Autodesk Fusion 360 part; units mm, degrees
(part 6 of 6)
  spline S11 degree 5 poles (-54.7383, -24.4894) (-54.7257, -24.481) (-54.7005, -24.464) (-54.6628, -24.4385) (-54.6128, -24.4043) (-54.5506, -24.3613) (-54.4888, -24.3181) (-54.4272, -24.2746) (-54.366, -24.2308) (-54.3052, -24.1868) (-54.2446, -24.1425) (-54.1845, -24.098) (-54.1246, -24.0531) (-54.0651, -24.0081) (-54.006, -23.9627) (-53.9472, -23.9171) (-53.8888, -23.8713) (-53.8308, -23.8252) (-53.7731, -23.7788) (-53.7158, -23.7322) (-53.6588, -23.6853) (-53.6023, -23.6381) (-53.5461, -23.5907) (-53.4903, -23.543) (-53.4349, -23.4951) (-53.3798, -23.4469) (-53.3252, -23.3985) (-53.271, -23.3498) (-53.2171, -23.3008) (-53.1637, -23.2516) (-53.1107, -23.2021) (-53.0581, -23.1524) (-53.006, -23.1024) (-52.9543, -23.0522) (-52.903, -23.0017) (-52.8521, -22.9509) (-52.8017, -22.8999) (-52.7517, -22.8486) (-52.7022, -22.797) (-52.6531, -22.7452) (-52.6046, -22.6931) (-52.5565, -22.6408) (-52.5088, -22.5882) (-52.4617, -22.5353) (-52.4151, -22.4822) (-52.369, -22.4288) (-52.3234, -22.3751) (-52.2783, -22.3212) (-52.2337, -22.267) (-52.1896, -22.2126) (-52.1461, -22.1579) (-52.1033, -22.1028) (-52.061, -22.0475) (-52.0194, -21.9919) (-51.9783, -21.936) (-51.9379, -21.8799) (-51.8981, -21.8234) (-51.8587, -21.7667) (-51.82, -21.7098) (-51.782, -21.6526) (-51.7447, -21.595) (-51.7084, -21.537) (-51.6732, -21.4786) (-51.6389, -21.4198) (-51.6056, -21.3607) (-51.5729, -21.3012) (-51.5407, -21.2416) (-51.5091, -21.1818) (-51.4781, -21.1218) (-51.4485, -21.0613) (-51.421, -21) (-51.4013, -20.9502) (-51.3882, -20.9122) (-51.3802, -20.8866) (-51.3764, -20.8737) knots -1 -1 -1 -1 -1 -1 -0.98571429 -0.97142857 -0.95714286 -0.94285714 -0.92857143 -0.91428571 -0.9 -0.88571429 -0.87142857 -0.85714286 -0.84285714 -0.82857143 -0.81428571 -0.8 -0.78571429 -0.77142857 -0.75714286 -0.74285714 -0.72857143 -0.71428571 -0.7 -0.68571429 -0.67142857 -0.65714286 -0.64285714 -0.62857143 -0.61428571 -0.6 -0.58571429 -0.57142857 -0.55714286 -0.54285714 -0.52857143 -0.51428571 -0.5 -0.48571429 -0.47142857 -0.45714286 -0.44285714 -0.42857143 -0.41428571 -0.4 -0.38571429 -0.37142857 -0.35714286 -0.34285714 -0.32857143 -0.31428571 -0.3 -0.28571429 -0.27142857 -0.25714286 -0.24285714 -0.22857143 -0.21428571 -0.2 -0.18571429 -0.17142857 -0.15714286 -0.14285714 -0.12857143 -0.11428571 -0.1 -0.08571429 -0.07142857 -0.05714286 -0.04285714 -0.02857143 -0.01428571 0 0 0 0 0 0
  line L13 (-51.3764, -20.8737) -> (-51.0935, -19.9176)
  arc A22 (-49.2442, -18.8145) -> (-51.0935, -19.9176) centre (-49.5712, -20.368) ccw
  arc A23 (-49.2442, -18.8145) -> (-48.5053, -18.9543) centre (-45.4614, -0.8441) ccw
  arc A24 (-47.1869, -20.6568) -> (-48.5053, -18.9543) centre (-48.7685, -20.5199) ccw
  line L14 (-47.1869, -20.6568) -> (-47.2729, -21.6501)
  spline S12 degree 5 poles (-47.2729, -21.6501) (-47.274, -21.6635) (-47.2759, -21.6902) (-47.2776, -21.7304) (-47.2775, -21.784) (-47.2743, -21.8511) (-47.2688, -21.9182) (-47.2619, -21.9854) (-47.2543, -22.0527) (-47.2461, -22.1199) (-47.2375, -22.1872) (-47.228, -22.2544) (-47.2176, -22.3217) (-47.2061, -22.3889) (-47.1935, -22.4561) (-47.1799, -22.5233) (-47.1654, -22.5905) (-47.1501, -22.6577) (-47.1342, -22.7248) (-47.1177, -22.7919) (-47.1006, -22.8589) (-47.0829, -22.9259) (-47.0644, -22.9929) (-47.0453, -23.0599) (-47.0255, -23.1267) (-47.005, -23.1936) (-46.9839, -23.2604) (-46.9622, -23.3271) (-46.9399, -23.3938) (-46.917, -23.4604) (-46.8936, -23.5269) (-46.8696, -23.5934) (-46.8451, -23.6598) (-46.82, -23.7262) (-46.7943, -23.7925) (-46.7681, -23.8587) (-46.7414, -23.9249) (-46.7141, -23.9909) (-46.6863, -24.0569) (-46.658, -24.1229) (-46.6292, -24.1887) (-46.5999, -24.2545) (-46.5702, -24.3201) (-46.5399, -24.3857) (-46.5091, -24.4512) (-46.4778, -24.5167) (-46.4461, -24.582) (-46.4139, -24.6472) (-46.3812, -24.7124) (-46.348, -24.7774) (-46.3144, -24.8424) (-46.2803, -24.9072) (-46.2458, -24.972) (-46.2108, -25.0367) (-46.1754, -25.1012) (-46.1395, -25.1657) (-46.1032, -25.23) (-46.0664, -25.2943) (-46.0292, -25.3584) (-45.9916, -25.4224) (-45.9536, -25.4863) (-45.9151, -25.5501) (-45.8762, -25.6138) (-45.8369, -25.6774) (-45.7971, -25.7409) (-45.757, -25.8042) (-45.7164, -25.8674) (-45.6754, -25.9305) (-45.634, -25.9935) (-45.5922, -26.0564) (-45.55, -26.1191) (-45.516, -26.1692) (-45.4902, -26.2067) (-45.473, -26.2317) (-45.4643, -26.2441) knots 0 0 0 0 0 0 0.01428571 0.02857143 0.04285714 0.05714286 0.07142857 0.08571429 0.1 0.11428571 0.12857143 0.14285714 0.15714286 0.17142857 0.18571429 0.2 0.21428571 0.22857143 0.24285714 0.25714286 0.27142857 0.28571429 0.3 0.31428571 0.32857143 0.34285714 0.35714286 0.37142857 0.38571429 0.4 0.41428571 0.42857143 0.44285714 0.45714286 0.47142857 0.48571429 0.5 0.51428571 0.52857143 0.54285714 0.55714286 0.57142857 0.58571429 0.6 0.61428571 0.62857143 0.64285714 0.65714286 0.67142857 0.68571429 0.7 0.71428571 0.72857143 0.74285714 0.75714286 0.77142857 0.78571429 0.8 0.81428571 0.82857143 0.84285714 0.85714286 0.87142857 0.88571429 0.9 0.91428571 0.92857143 0.94285714 0.95714286 0.97142857 0.98571429 1 1 1 1 1 1
  arc A25 (-45.4643, -26.2441) -> (-43.5603, -26.1729) centre (-45.4614, -0.8441) ccw
  spline S13 degree 5 poles (-43.5603, -26.1729) (-43.5526, -26.1598) (-43.5373, -26.1336) (-43.5144, -26.0943) (-43.4842, -26.0418) (-43.4468, -25.9761) (-43.4098, -25.9103) (-43.3732, -25.8444) (-43.3371, -25.7784) (-43.3013, -25.7123) (-43.266, -25.6462) (-43.2311, -25.5799) (-43.1967, -25.5136) (-43.1626, -25.4471) (-43.129, -25.3806) (-43.0959, -25.3141) (-43.0631, -25.2474) (-43.0308, -25.1807) (-42.999, -25.1139) (-42.9676, -25.047) (-42.9366, -24.98) (-42.9061, -24.913) (-42.8761, -24.8459) (-42.8465, -24.7788) (-42.8173, -24.7115) (-42.7887, -24.6442) (-42.7605, -24.5769) (-42.7327, -24.5095) (-42.7055, -24.442) (-42.6787, -24.3745) (-42.6524, -24.3069) (-42.6266, -24.2393) (-42.6013, -24.1716) (-42.5765, -24.1039) (-42.5522, -24.0362) (-42.5284, -23.9683) (-42.5052, -23.9005) (-42.4824, -23.8326) (-42.4601, -23.7647) (-42.4384, -23.6967) (-42.4172, -23.6287) (-42.3966, -23.5607) (-42.3765, -23.4926) (-42.357, -23.4246) (-42.3381, -23.3565) (-42.3197, -23.2884) (-42.3019, -23.2202) (-42.2846, -23.1521) (-42.268, -23.0839) (-42.2519, -23.0157) (-42.2365, -22.9475) (-42.2217, -22.8794) (-42.2076, -22.8112) (-42.1942, -22.743) (-42.1815, -22.6749) (-42.1695, -22.6067) (-42.1581, -22.5386) (-42.1472, -22.4705) (-42.137, -22.4024) (-42.1276, -22.3343) (-42.119, -22.2663) (-42.1115, -22.1983) (-42.105, -22.1304) (-42.0997, -22.0625) (-42.0953, -21.9948) (-42.0917, -21.927) (-42.0886, -21.8594) (-42.086, -21.7918) (-42.0841, -21.7242) (-42.0837, -21.6569) (-42.0855, -21.5897) (-42.0894, -21.5363) (-42.0941, -21.4963) (-42.098, -21.4698) (-42.1001, -21.4566) knots -1 -1 -1 -1 -1 -1 -0.98571429 -0.97142857 -0.95714286 -0.94285714 -0.92857143 -0.91428571 -0.9 -0.88571429 -0.87142857 -0.85714286 -0.84285714 -0.82857143 -0.81428571 -0.8 -0.78571429 -0.77142857 -0.75714286 -0.74285714 -0.72857143 -0.71428571 -0.7 -0.68571429 -0.67142857 -0.65714286 -0.64285714 -0.62857143 -0.61428571 -0.6 -0.58571429 -0.57142857 -0.55714286 -0.54285714 -0.52857143 -0.51428571 -0.5 -0.48571429 -0.47142857 -0.45714286 -0.44285714 -0.42857143 -0.41428571 -0.4 -0.38571429 -0.37142857 -0.35714286 -0.34285714 -0.32857143 -0.31428571 -0.3 -0.28571429 -0.27142857 -0.25714286 -0.24285714 -0.22857143 -0.21428571 -0.2 -0.18571429 -0.17142857 -0.15714286 -0.14285714 -0.12857143 -0.11428571 -0.1 -0.08571429 -0.07142857 -0.05714286 -0.04285714 -0.02857143 -0.01428571 0 0 0 0 0 0
  line L15 (-42.1001, -21.4566) -> (-42.2601, -20.4724)
  arc A26 (-41.0726, -18.6762) -> (-42.2601, -20.4724) centre (-40.6932, -20.2177) ccw
  arc A27 (-41.0726, -18.6762) -> (-40.3462, -18.4816) centre (-45.4614, -0.8441) ccw
  arc A28 (-38.4196, -19.4434) -> (-40.3462, -18.4816) centre (-39.904, -20.0062) ccw
  line L16 (-38.4196, -19.4434) -> (-38.0661, -20.3756)
  spline S14 degree 5 poles (-38.0661, -20.3756) (-38.0613, -20.3882) (-38.0515, -20.4131) (-38.0355, -20.45) (-38.0122, -20.4983) (-37.9802, -20.5573) (-37.9461, -20.6155) (-37.9108, -20.673) (-37.8747, -20.7303) (-37.8382, -20.7873) (-37.8012, -20.8441) (-37.7635, -20.9006) (-37.725, -20.9567) (-37.6854, -21.0123) (-37.6449, -21.0674) (-37.6034, -21.122) (-37.5612, -21.1763) (-37.5183, -21.2302) (-37.4749, -21.2837) (-37.4309, -21.337) (-37.3864, -21.39) (-37.3414, -21.4427) (-37.2957, -21.495) (-37.2494, -21.547) (-37.2025, -21.5987) (-37.1551, -21.65) (-37.1071, -21.701) (-37.0586, -21.7517) (-37.0095, -21.8021) (-36.96, -21.8522) (-36.9101, -21.902) (-36.8596, -21.9515) (-36.8087, -22.0007) (-36.7573, -22.0496) (-36.7054, -22.0982) (-36.653, -22.1465) (-36.6003, -22.1945) (-36.547, -22.2422) (-36.4934, -22.2896) (-36.4393, -22.3368) (-36.3848, -22.3836) (-36.3298, -22.4301) (-36.2745, -22.4764) (-36.2187, -22.5223) (-36.1626, -22.568) (-36.106, -22.6134) (-36.0491, -22.6585) (-35.9918, -22.7033) (-35.9341, -22.7478) (-35.876, -22.792) (-35.8175, -22.8359) (-35.7586, -22.8796) (-35.6994, -22.9229) (-35.6399, -22.966) (-35.5799, -23.0088) (-35.5196, -23.0513) (-35.459, -23.0935) (-35.398, -23.1355) (-35.3367, -23.1771) (-35.275, -23.2185) (-35.213, -23.2595) (-35.1506, -23.3003) (-35.0879, -23.3408) (-35.0249, -23.3811) (-34.9616, -23.421) (-34.8979, -23.4606) (-34.8339, -23.5) (-34.7696, -23.5391) (-34.705, -23.5778) (-34.6401, -23.6163) (-34.5749, -23.6545) (-34.5224, -23.6849) (-34.483, -23.7075) (-34.4566, -23.7225) (-34.4434, -23.73) knots 0 0 0 0 0 0 0.01428571 0.02857143 0.04285714 0.05714286 0.07142857 0.08571429 0.1 0.11428571 0.12857143 0.14285714 0.15714286 0.17142857 0.18571429 0.2 0.21428571 0.22857143 0.24285714 0.25714286 0.27142857 0.28571429 0.3 0.31428571 0.32857143 0.34285714 0.35714286 0.37142857 0.38571429 0.4 0.41428571 0.42857143 0.44285714 0.45714286 0.47142857 0.48571429 0.5 0.51428571 0.52857143 0.54285714 0.55714286 0.57142857 0.58571429 0.6 0.61428571 0.62857143 0.64285714 0.65714286 0.67142857 0.68571429 0.7 0.71428571 0.72857143 0.74285714 0.75714286 0.77142857 0.78571429 0.8 0.81428571 0.82857143 0.84285714 0.85714286 0.87142857 0.88571429 0.9 0.91428571 0.92857143 0.94285714 0.95714286 0.97142857 0.98571429 1 1 1 1 1 1
  arc A29 (-34.4434, -23.73) -> (-32.7588, -22.8397) centre (-45.4614, -0.8441) ccw
  spline S15 degree 5 poles (-32.7588, -22.8397) (-32.7576, -22.8246) (-32.7551, -22.7943) (-32.7516, -22.749) (-32.7471, -22.6886) (-32.7419, -22.6131) (-32.7372, -22.5378) (-32.7328, -22.4626) (-32.7289, -22.3874) (-32.7254, -22.3124) (-32.7223, -22.2375) (-32.7196, -22.1626) (-32.7173, -22.0879) (-32.7154, -22.0133) (-32.714, -21.9388) (-32.713, -21.8644) (-32.7125, -21.7902) (-32.7123, -21.716) (-32.7126, -21.642) (-32.7133, -21.5681) (-32.7145, -21.4944) (-32.7161, -21.4208) (-32.7181, -21.3473) (-32.7206, -21.2739) (-32.7235, -21.2007) (-32.7269, -21.1277) (-32.7307, -21.0547) (-32.735, -20.982) (-32.7397, -20.9094) (-32.7448, -20.8369) (-32.7505, -20.7646) (-32.7566, -20.6925) (-32.7631, -20.6206) (-32.7702, -20.5488) (-32.7777, -20.4772) (-32.7857, -20.4058) (-32.7941, -20.3345) (-32.8031, -20.2635) (-32.8125, -20.1926) (-32.8224, -20.122) (-32.8328, -20.0515) (-32.8438, -19.9813) (-32.8552, -19.9113) (-32.8672, -19.8415) (-32.8796, -19.7719) (-32.8926, -19.7026) (-32.9062, -19.6334) (-32.9202, -19.5646) (-32.9347, -19.4959) (-32.9499, -19.4275) (-32.9655, -19.3594) (-32.9818, -19.2916) (-32.9987, -19.224) (-33.0162, -19.1568) (-33.0343, -19.0899) (-33.0531, -19.0233) (-33.0723, -18.9569) (-33.0921, -18.8908) (-33.1125, -18.8251) (-33.1335, -18.7596) (-33.1553, -18.6946) (-33.178, -18.6301) (-33.2017, -18.5661) (-33.2263, -18.5027) (-33.2517, -18.4397) (-33.2778, -18.3771) (-33.3044, -18.3148) (-33.3314, -18.2528) (-33.3591, -18.1911) (-33.3879, -18.1302) (-33.4186, -18.0705) (-33.4453, -18.0241) (-33.4669, -17.9901) (-33.4819, -17.9679) (-33.4896, -17.9569) knots -1 -1 -1 -1 -1 -1 -0.98571429 -0.97142857 -0.95714286 -0.94285714 -0.92857143 -0.91428571 -0.9 -0.88571429 -0.87142857 -0.85714286 -0.84285714 -0.82857143 -0.81428571 -0.8 -0.78571429 -0.77142857 -0.75714286 -0.74285714 -0.72857143 -0.71428571 -0.7 -0.68571429 -0.67142857 -0.65714286 -0.64285714 -0.62857143 -0.61428571 -0.6 -0.58571429 -0.57142857 -0.55714286 -0.54285714 -0.52857143 -0.51428571 -0.5 -0.48571429 -0.47142857 -0.45714286 -0.44285714 -0.42857143 -0.41428571 -0.4 -0.38571429 -0.37142857 -0.35714286 -0.34285714 -0.32857143 -0.31428571 -0.3 -0.28571429 -0.27142857 -0.25714286 -0.24285714 -0.22857143 -0.21428571 -0.2 -0.18571429 -0.17142857 -0.15714286 -0.14285714 -0.12857143 -0.11428571 -0.1 -0.08571429 -0.07142857 -0.05714286 -0.04285714 -0.02857143 -0.01428571 0 0 0 0 0 0
  line L17 (-33.4896, -17.9569) -> (-34.0607, -17.1396)
  arc A30 (-33.7702, -15.006) -> (-34.0607, -17.1396) centre (-32.7595, -16.2303) ccw
  arc A31 (-33.7702, -15.006) -> (-33.2001, -14.5155) centre (-45.4614, -0.8441) ccw
  arc A32 (-31.0471, -14.5462) -> (-33.2001, -14.5155) centre (-32.1402, -15.6973) ccw
  line L18 (-31.0471, -14.5462) -> (-30.3241, -15.2327)
  spline S16 degree 5 poles (-30.3241, -15.2327) (-30.3143, -15.242) (-30.2946, -15.2602) (-30.2642, -15.2865) (-30.2223, -15.3199) (-30.1678, -15.3592) (-30.1119, -15.3967) (-30.0551, -15.4332) (-29.9978, -15.4692) (-29.9401, -15.5048) (-29.8821, -15.5399) (-29.8236, -15.5744) (-29.7646, -15.6082) (-29.7048, -15.6412) (-29.6444, -15.6732) (-29.5834, -15.7045) (-29.5218, -15.735) (-29.4598, -15.765) (-29.3974, -15.7944) (-29.3347, -15.8233) (-29.2716, -15.8518) (-29.2081, -15.8797) (-29.1443, -15.907) (-29.08, -15.9338) (-29.0153, -15.96) (-28.9503, -15.9856) (-28.8849, -16.0108) (-28.8192, -16.0354) (-28.7532, -16.0595) (-28.6869, -16.0832) (-28.6202, -16.1064) (-28.5533, -16.1291) (-28.4861, -16.1513) (-28.4185, -16.1731) (-28.3507, -16.1943) (-28.2826, -16.2151) (-28.2142, -16.2355) (-28.1455, -16.2554) (-28.0766, -16.2748) (-28.0074, -16.2938) (-27.938, -16.3123) (-27.8683, -16.3304) (-27.7984, -16.3481) (-27.7282, -16.3653) (-27.6578, -16.3821) (-27.5872, -16.3984) (-27.5163, -16.4143) (-27.4452, -16.4298) (-27.3739, -16.4449) (-27.3024, -16.4595) (-27.2307, -16.4737) (-27.1587, -16.4875) (-27.0865, -16.5009) (-27.0142, -16.5139) (-26.9416, -16.5264) (-26.8689, -16.5386) (-26.7959, -16.5503) (-26.7228, -16.5616) (-26.6494, -16.5725) (-26.5759, -16.583) (-26.5022, -16.5931) (-26.4283, -16.6028) (-26.3543, -16.6121) (-26.2801, -16.621) (-26.2057, -16.6295) (-26.1311, -16.6376) (-26.0564, -16.6453) (-25.9815, -16.6526) (-25.9065, -16.6595) (-25.8313, -16.666) (-25.7559, -16.6721) (-25.6955, -16.6767) (-25.6501, -16.68) (-25.6199, -16.6821) (-25.6047, -16.6831) knots 0 0 0 0 0 0 0.01428571 0.02857143 0.04285714 0.05714286 0.07142857 0.08571429 0.1 0.11428571 0.12857143 0.14285714 0.15714286 0.17142857 0.18571429 0.2 0.21428571 0.22857143 0.24285714 0.25714286 0.27142857 0.28571429 0.3 0.31428571 0.32857143 0.34285714 0.35714286 0.37142857 0.38571429 0.4 0.41428571 0.42857143 0.44285714 0.45714286 0.47142857 0.48571429 0.5 0.51428571 0.52857143 0.54285714 0.55714286 0.57142857 0.58571429 0.6 0.61428571 0.62857143 0.64285714 0.65714286 0.67142857 0.68571429 0.7 0.71428571 0.72857143 0.74285714 0.75714286 0.77142857 0.78571429 0.8 0.81428571 0.82857143 0.84285714 0.85714286 0.87142857 0.88571429 0.9 0.91428571 0.92857143 0.94285714 0.95714286 0.97142857 0.98571429 1 1 1 1 1 1
  arc A33 (-25.6047, -16.6831) -> (-24.4732, -15.15) centre (-45.4614, -0.8441) ccw
  spline S17 degree 5 poles (-24.4732, -15.15) (-24.4787, -15.1359) (-24.4896, -15.1075) (-24.5061, -15.0651) (-24.5283, -15.0088) (-24.5564, -14.9386) (-24.5847, -14.8686) (-24.6135, -14.799) (-24.6425, -14.7296) (-24.6719, -14.6604) (-24.7016, -14.5916) (-24.7317, -14.523) (-24.762, -14.4547) (-24.7927, -14.3866) (-24.8238, -14.3189) (-24.8552, -14.2515) (-24.8869, -14.1843) (-24.9189, -14.1175) (-24.9513, -14.0509) (-24.984, -13.9846) (-25.017, -13.9187) (-25.0504, -13.8531) (-25.0841, -13.7877) (-25.1182, -13.7227) (-25.1526, -13.658) (-25.1873, -13.5937) (-25.2224, -13.5296) (-25.2578, -13.4659) (-25.2935, -13.4025) (-25.3296, -13.3395) (-25.3661, -13.2768) (-25.4029, -13.2145) (-25.44, -13.1525) (-25.4775, -13.0909) (-25.5153, -13.0297) (-25.5535, -12.9688) (-25.592, -12.9083) (-25.6309, -12.8481) (-25.6701, -12.7884) (-25.7097, -12.729) (-25.7497, -12.6701) (-25.79, -12.6115) (-25.8307, -12.5534) (-25.8718, -12.4957) (-25.9132, -12.4385) (-25.955, -12.3816) (-25.9971, -12.3252) (-26.0397, -12.2692) (-26.0826, -12.2137) (-26.1259, -12.1586) (-26.1695, -12.1041) (-26.2136, -12.05) (-26.2582, -11.9965) (-26.3031, -11.9435) (-26.3485, -11.8911) (-26.3942, -11.8392) (-26.4404, -11.7878) (-26.4869, -11.7368) (-26.5338, -11.6864) (-26.5811, -11.6366) (-26.629, -11.5875) (-26.6774, -11.5392) (-26.7265, -11.4918) (-26.7762, -11.4453) (-26.8265, -11.3996) (-26.8771, -11.3546) (-26.9281, -11.3099) (-26.9793, -11.2658) (-27.031, -11.2222) (-27.0834, -11.1799) (-27.137, -11.1394) (-27.1812, -11.1092) (-27.2153, -11.0879) (-27.2385, -11.0744) (-27.2502, -11.0678) knots -1 -1 -1 -1 -1 -1 -0.98571429 -0.97142857 -0.95714286 -0.94285714 -0.92857143 -0.91428571 -0.9 -0.88571429 -0.87142857 -0.85714286 -0.84285714 -0.82857143 -0.81428571 -0.8 -0.78571429 -0.77142857 -0.75714286 -0.74285714 -0.72857143 -0.71428571 -0.7 -0.68571429 -0.67142857 -0.65714286 -0.64285714 -0.62857143 -0.61428571 -0.6 -0.58571429 -0.57142857 -0.55714286 -0.54285714 -0.52857143 -0.51428571 -0.5 -0.48571429 -0.47142857 -0.45714286 -0.44285714 -0.42857143 -0.41428571 -0.4 -0.38571429 -0.37142857 -0.35714286 -0.34285714 -0.32857143 -0.31428571 -0.3 -0.28571429 -0.27142857 -0.25714286 -0.24285714 -0.22857143 -0.21428571 -0.2 -0.18571429 -0.17142857 -0.15714286 -0.14285714 -0.12857143 -0.11428571 -0.1 -0.08571429 -0.07142857 -0.05714286 -0.04285714 -0.02857143 -0.01428571 0 0 0 0 0 0
  line L19 (-27.2502, -11.0678) -> (-28.1194, -10.5793)
  arc A34 (-28.7833, -8.5309) -> (-28.1194, -10.5793) centre (-27.3416, -9.1954) ccw
  arc A35 (-28.7833, -8.5309) -> (-28.4826, -7.8417) centre (-45.4614, -0.8441) ccw
  arc A36 (-26.5294, -6.9351) -> (-28.4826, -7.8417) centre (-27.0149, -8.4466) ccw
  line L20 (-26.5294, -6.9351) -> (-25.5802, -7.24)
  spline S18 degree 5 poles (-25.5802, -7.24) (-25.5674, -7.2441) (-25.5417, -7.2519) (-25.5029, -7.2625) (-25.4506, -7.2743) (-25.3845, -7.2861) (-25.3178, -7.2957) (-25.2508, -7.3039) (-25.1836, -7.3115) (-25.1162, -7.3185) (-25.0487, -7.325) (-24.981, -7.3307) (-24.9131, -7.3356) (-24.845, -7.3393) (-24.7767, -7.342) (-24.7081, -7.3436) (-24.6394, -7.3444) (-24.5705, -7.3445) (-24.5016, -7.344) (-24.4325, -7.3428) (-24.3633, -7.3411) (-24.294, -7.3387) (-24.2246, -7.3356) (-24.1551, -7.3318) (-24.0855, -7.3274) (-24.0158, -7.3223) (-23.946, -7.3165) (-23.8761, -7.3102) (-23.8061, -7.3033) (-23.7361, -7.2959) (-23.666, -7.2878) (-23.5958, -7.2793) (-23.5256, -7.2701) (-23.4553, -7.2604) (-23.385, -7.2501) (-23.3146, -7.2393) (-23.2442, -7.228) (-23.1737, -7.2161) (-23.1031, -7.2037) (-23.0326, -7.1908) (-22.962, -7.1774) (-22.8914, -7.1635) (-22.8207, -7.149) (-22.75, -7.1341) (-22.6793, -7.1187) (-22.6086, -7.1027) (-22.5378, -7.0863) (-22.467, -7.0694) (-22.3962, -7.0521) (-22.3254, -7.0342) (-22.2546, -7.0159) (-22.1838, -6.9971) (-22.113, -6.9779) (-22.0422, -6.9581) (-21.9714, -6.938) (-21.9005, -6.9173) (-21.8297, -6.8962) (-21.7589, -6.8747) (-21.6881, -6.8527) (-21.6173, -6.8303) (-21.5465, -6.8074) (-21.4758, -6.7841) (-21.405, -6.7603) (-21.3343, -6.7361) (-21.2636, -6.7115) (-21.1929, -6.6865) (-21.1222, -6.661) (-21.0516, -6.6351) (-20.981, -6.6087) (-20.9104, -6.582) (-20.8399, -6.5548) (-20.7834, -6.5327) (-20.7412, -6.516) (-20.713, -6.5047) (-20.6989, -6.4991) knots 0 0 0 0 0 0 0.01428571 0.02857143 0.04285714 0.05714286 0.07142857 0.08571429 0.1 0.11428571 0.12857143 0.14285714 0.15714286 0.17142857 0.18571429 0.2 0.21428571 0.22857143 0.24285714 0.25714286 0.27142857 0.28571429 0.3 0.31428571 0.32857143 0.34285714 0.35714286 0.37142857 0.38571429 0.4 0.41428571 0.42857143 0.44285714 0.45714286 0.47142857 0.48571429 0.5 0.51428571 0.52857143 0.54285714 0.55714286 0.57142857 0.58571429 0.6 0.61428571 0.62857143 0.64285714 0.65714286 0.67142857 0.68571429 0.7 0.71428571 0.72857143 0.74285714 0.75714286 0.77142857 0.78571429 0.8 0.81428571 0.82857143 0.84285714 0.85714286 0.87142857 0.88571429 0.9 0.91428571 0.92857143 0.94285714 0.95714286 0.97142857 0.98571429 1 1 1 1 1 1
  arc A37 (-20.6989, -6.4991) -> (-20.3446, -4.6269) centre (-45.4614, -0.8441) ccw
  spline S19 degree 5 poles (-20.3446, -4.6269) (-20.3557, -4.6165) (-20.3778, -4.5957) (-20.4111, -4.5647) (-20.4555, -4.5235) (-20.5113, -4.4724) (-20.5672, -4.4217) (-20.6233, -4.3714) (-20.6796, -4.3215) (-20.736, -4.272) (-20.7927, -4.2228) (-20.8495, -4.1741) (-20.9065, -4.1257) (-20.9637, -4.0777) (-21.0211, -4.0302) (-21.0786, -3.983) (-21.1363, -3.9363) (-21.1942, -3.8899) (-21.2522, -3.844) (-21.3104, -3.7985) (-21.3688, -3.7534) (-21.4274, -3.7088) (-21.4861, -3.6645) (-21.545, -3.6208) (-21.604, -3.5774) (-21.6633, -3.5345) (-21.7226, -3.492) (-21.7822, -3.45) (-21.8419, -3.4084) (-21.9018, -3.3673) (-21.9618, -3.3266) (-22.022, -3.2864) (-22.0823, -3.2467) (-22.1428, -3.2074) (-22.2035, -3.1686) (-22.2643, -3.1304) (-22.3253, -3.0926) (-22.3864, -3.0553) (-22.4477, -3.0185) (-22.5091, -2.9822) (-22.5707, -2.9464) (-22.6324, -2.9111) (-22.6943, -2.8764) (-22.7563, -2.8422) (-22.8185, -2.8086) (-22.8808, -2.7755) (-22.9433, -2.743) (-23.0059, -2.711) (-23.0686, -2.6796) (-23.1315, -2.6488) (-23.1945, -2.6186) (-23.2577, -2.589) (-23.3211, -2.5601) (-23.3845, -2.5319) (-23.4482, -2.5043) (-23.5119, -2.4774) (-23.5758, -2.4511) (-23.6398, -2.4254) (-23.7039, -2.4003) (-23.7682, -2.376) (-23.8326, -2.3525) (-23.8972, -2.33) (-23.962, -2.3086) (-24.0269, -2.2883) (-24.092, -2.2689) (-24.1572, -2.2503) (-24.2225, -2.2322) (-24.2879, -2.2147) (-24.3533, -2.1978) (-24.4189, -2.1824) (-24.4847, -2.1692) (-24.5377, -2.1611) (-24.5777, -2.1568) (-24.6044, -2.1547) (-24.6178, -2.1539) knots -1 -1 -1 -1 -1 -1 -0.98571429 -0.97142857 -0.95714286 -0.94285714 -0.92857143 -0.91428571 -0.9 -0.88571429 -0.87142857 -0.85714286 -0.84285714 -0.82857143 -0.81428571 -0.8 -0.78571429 -0.77142857 -0.75714286 -0.74285714 -0.72857143 -0.71428571 -0.7 -0.68571429 -0.67142857 -0.65714286 -0.64285714 -0.62857143 -0.61428571 -0.6 -0.58571429 -0.57142857 -0.55714286 -0.54285714 -0.52857143 -0.51428571 -0.5 -0.48571429 -0.47142857 -0.45714286 -0.44285714 -0.42857143 -0.41428571 -0.4 -0.38571429 -0.37142857 -0.35714286 -0.34285714 -0.32857143 -0.31428571 -0.3 -0.28571429 -0.27142857 -0.25714286 -0.24285714 -0.22857143 -0.21428571 -0.2 -0.18571429 -0.17142857 -0.15714286 -0.14285714 -0.12857143 -0.11428571 -0.1 -0.08571429 -0.07142857 -0.05714286 -0.04285714 -0.02857143 -0.01428571 0 0 0 0 0 0
  line L21 (-24.6178, -2.1539) -> (-25.6129, -2.0908)
  arc A38 (-27.0998, -0.5334) -> (-25.6129, -2.0908) centre (-25.5125, -0.5065) ccw
  arc A39 (-27.0998, -0.5334) -> (-27.1279, 0.2181) centre (-45.4614, -0.8441) ccw
  arc A40 (-25.7615, 1.8823) -> (-27.1279, 0.2181) centre (-25.5431, 0.31) ccw
  line L22 (-25.7615, 1.8823) -> (-24.774, 2.0195)
  spline S20 degree 5 poles (-24.774, 2.0195) (-24.7607, 2.0214) (-24.7342, 2.0255) (-24.6946, 2.0328) (-24.6424, 2.0448) (-24.5777, 2.0629) (-24.5135, 2.0832) (-24.4495, 2.1048) (-24.3856, 2.1272) (-24.3219, 2.1501) (-24.2583, 2.1736) (-24.1948, 2.1977) (-24.1315, 2.2228) (-24.0685, 2.249) (-24.0058, 2.2763) (-23.9433, 2.3045) (-23.8811, 2.3336) (-23.819, 2.3634) (-23.7571, 2.3938) (-23.6953, 2.4248) (-23.6338, 2.4564) (-23.5724, 2.4887) (-23.5112, 2.5216) (-23.4502, 2.5551) (-23.3894, 2.5893) (-23.3288, 2.6242) (-23.2684, 2.6596) (-23.2082, 2.6956) (-23.1481, 2.7322) (-23.0883, 2.7693) (-23.0286, 2.8069) (-22.9691, 2.8451) (-22.9098, 2.8838) (-22.8507, 2.9231) (-22.7918, 2.9628) (-22.7331, 3.0031) (-22.6745, 3.0439) (-22.6162, 3.0852) (-22.558, 3.127) (-22.5, 3.1692) (-22.4422, 3.2119) (-22.3846, 3.2551) (-22.3272, 3.2988) (-22.27, 3.3429) (-22.213, 3.3875) (-22.1562, 3.4325) (-22.0996, 3.478) (-22.0431, 3.5239) (-21.9869, 3.5703) (-21.9309, 3.6171) (-21.875, 3.6643) (-21.8194, 3.712) (-21.7639, 3.76) (-21.7086, 3.8085) (-21.6536, 3.8574) (-21.5987, 3.9068) (-21.5441, 3.9565) (-21.4896, 4.0066) (-21.4354, 4.0572) (-21.3813, 4.1081) (-21.3275, 4.1594) (-21.2739, 4.2111) (-21.2204, 4.2632) (-21.1672, 4.3157) (-21.1142, 4.3686) (-21.0613, 4.4218) (-21.0087, 4.4754) (-20.9563, 4.5294) (-20.9041, 4.5838) (-20.8522, 4.6385) (-20.8004, 4.6936) (-20.7592, 4.738) (-20.7283, 4.7714) (-20.7078, 4.7938) (-20.6975, 4.805) knots 0 0 0 0 0 0 0.01428571 0.02857143 0.04285714 0.05714286 0.07142857 0.08571429 0.1 0.11428571 0.12857143 0.14285714 0.15714286 0.17142857 0.18571429 0.2 0.21428571 0.22857143 0.24285714 0.25714286 0.27142857 0.28571429 0.3 0.31428571 0.32857143 0.34285714 0.35714286 0.37142857 0.38571429 0.4 0.41428571 0.42857143 0.44285714 0.45714286 0.47142857 0.48571429 0.5 0.51428571 0.52857143 0.54285714 0.55714286 0.57142857 0.58571429 0.6 0.61428571 0.62857143 0.64285714 0.65714286 0.67142857 0.68571429 0.7 0.71428571 0.72857143 0.74285714 0.75714286 0.77142857 0.78571429 0.8 0.81428571 0.82857143 0.84285714 0.85714286 0.87142857 0.88571429 0.9 0.91428571 0.92857143 0.94285714 0.95714286 0.97142857 0.98571429 1 1 1 1 1 1
  arc A41 (-20.6975, 4.805) -> (-21.1907, 6.6455) centre (-45.4614, -0.8441) ccw
  spline S21 degree 5 poles (-21.1907, 6.6455) (-21.2052, 6.65) (-21.2341, 6.6592) (-21.2776, 6.6727) (-21.3355, 6.6905) (-21.4078, 6.7123) (-21.4802, 6.7337) (-21.5526, 6.7547) (-21.625, 6.7753) (-21.6974, 6.7954) (-21.7697, 6.8151) (-21.8421, 6.8344) (-21.9144, 6.8532) (-21.9867, 6.8716) (-22.059, 6.8896) (-22.1313, 6.9071) (-22.2036, 6.9242) (-22.2759, 6.9408) (-22.3481, 6.957) (-22.4203, 6.9728) (-22.4924, 6.988) (-22.5646, 7.0029) (-22.6367, 7.0172) (-22.7087, 7.0312) (-22.7807, 7.0446) (-22.8527, 7.0576) (-22.9247, 7.0701) (-22.9965, 7.0821) (-23.0684, 7.0937) (-23.1402, 7.1047) (-23.2119, 7.1153) (-23.2836, 7.1254) (-23.3552, 7.135) (-23.4267, 7.1442) (-23.4982, 7.1528) (-23.5696, 7.1609) (-23.6409, 7.1685) (-23.7122, 7.1756) (-23.7833, 7.1821) (-23.8544, 7.1882) (-23.9254, 7.1937) (-23.9964, 7.1987) (-24.0672, 7.2031) (-24.1379, 7.207) (-24.2085, 7.2103) (-24.279, 7.2131) (-24.3494, 7.2153) (-24.4197, 7.2169) (-24.4898, 7.218) (-24.5599, 7.2185) (-24.6298, 7.2184) (-24.6995, 7.2176) (-24.7691, 7.2162) (-24.8385, 7.214) (-24.9078, 7.2113) (-24.9769, 7.2078) (-25.0459, 7.2038) (-25.1147, 7.1992) (-25.1834, 7.194) (-25.2519, 7.1881) (-25.3201, 7.1813) (-25.3881, 7.1735) (-25.4557, 7.1647) (-25.523, 7.1548) (-25.5901, 7.144) (-25.6569, 7.1325) (-25.7236, 7.1204) (-25.7901, 7.1079) (-25.8563, 7.0947) (-25.9221, 7.0801) (-25.9871, 7.0634) (-26.0384, 7.0477) (-26.0763, 7.0343) (-26.1013, 7.0246) (-26.1137, 7.0195) knots -1 -1 -1 -1 -1 -1 -0.98571429 -0.97142857 -0.95714286 -0.94285714 -0.92857143 -0.91428571 -0.9 -0.88571429 -0.87142857 -0.85714286 -0.84285714 -0.82857143 -0.81428571 -0.8 -0.78571429 -0.77142857 -0.75714286 -0.74285714 -0.72857143 -0.71428571 -0.7 -0.68571429 -0.67142857 -0.65714286 -0.64285714 -0.62857143 -0.61428571 -0.6 -0.58571429 -0.57142857 -0.55714286 -0.54285714 -0.52857143 -0.51428571 -0.5 -0.48571429 -0.47142857 -0.45714286 -0.44285714 -0.42857143 -0.41428571 -0.4 -0.38571429 -0.37142857 -0.35714286 -0.34285714 -0.32857143 -0.31428571 -0.3 -0.28571429 -0.27142857 -0.25714286 -0.24285714 -0.22857143 -0.21428571 -0.2 -0.18571429 -0.17142857 -0.15714286 -0.14285714 -0.12857143 -0.11428571 -0.1 -0.08571429 -0.07142857 -0.05714286 -0.04285714 -0.02857143 -0.01428571 0 0 0 0 0 0
  line L23 (-26.1137, 7.0195) -> (-27.0376, 6.6446)
  arc A42 (-29.053, 7.4026) -> (-27.0376, 6.6446) centre (-27.6346, 8.1155) ccw
  arc A43 (-29.053, 7.4026) -> (-29.4044, 8.0675) centre (-45.4614, -0.8441) ccw
  arc A44 (-28.8954, 10.1598) -> (-29.4044, 8.0675) centre (-28.0164, 8.8379) ccw
  line L24 (-28.8954, 10.1598) -> (-28.0652, 10.7119)
  spline S22 degree 5 poles (-28.0652, 10.7119) (-28.054, 10.7193) (-28.0319, 10.7345) (-27.9994, 10.7582) (-27.9576, 10.7917) (-27.9071, 10.8361) (-27.8581, 10.8822) (-27.8098, 10.9295) (-27.762, 10.9774) (-27.7145, 11.0257) (-27.6674, 11.0744) (-27.6207, 11.1237) (-27.5746, 11.1738) (-27.5292, 11.2247) (-27.4845, 11.2765) (-27.4404, 11.329) (-27.397, 11.3823) (-27.354, 11.4361) (-27.3114, 11.4903) (-27.2692, 11.545) (-27.2275, 11.6002) (-27.1861, 11.6559) (-27.1453, 11.7121) (-27.1049, 11.7688) (-27.0649, 11.826) (-27.0255, 11.8837) (-26.9864, 11.9418) (-26.9478, 12.0004) (-26.9096, 12.0594) (-26.8717, 12.1188) (-26.8343, 12.1786) (-26.7973, 12.2388) (-26.7606, 12.2994) (-26.7244, 12.3604) (-26.6886, 12.4218) (-26.6531, 12.4836) (-26.6181, 12.5457) (-26.5834, 12.6082) (-26.5491, 12.6711) (-26.5152, 12.7343) (-26.4817, 12.7979) (-26.4486, 12.8618) (-26.4158, 12.926) (-26.3834, 12.9906) (-26.3514, 13.0555) (-26.3197, 13.1207) (-26.2884, 13.1863) (-26.2575, 13.2522) (-26.227, 13.3183) (-26.1968, 13.3848) (-26.1669, 13.4516) (-26.1375, 13.5187) (-26.1084, 13.586) (-26.0796, 13.6537) (-26.0513, 13.7217) (-26.0232, 13.7899) (-25.9956, 13.8584) (-25.9683, 13.9272) (-25.9413, 13.9963) (-25.9147, 14.0656) (-25.8885, 14.1352) (-25.8626, 14.2051) (-25.837, 14.2752) (-25.8118, 14.3456) (-25.787, 14.4162) (-25.7625, 14.4871) (-25.7384, 14.5582) (-25.7146, 14.6296) (-25.6912, 14.7012) (-25.6681, 14.7731) (-25.6454, 14.8452) (-25.6274, 14.9031) (-25.6142, 14.9466) (-25.6054, 14.9756) (-25.601, 14.9902) knots 0 0 0 0 0 0 0.01428571 0.02857143 0.04285714 0.05714286 0.07142857 0.08571429 0.1 0.11428571 0.12857143 0.14285714 0.15714286 0.17142857 0.18571429 0.2 0.21428571 0.22857143 0.24285714 0.25714286 0.27142857 0.28571429 0.3 0.31428571 0.32857143 0.34285714 0.35714286 0.37142857 0.38571429 0.4 0.41428571 0.42857143 0.44285714 0.45714286 0.47142857 0.48571429 0.5 0.51428571 0.52857143 0.54285714 0.55714286 0.57142857 0.58571429 0.6 0.61428571 0.62857143 0.64285714 0.65714286 0.67142857 0.68571429 0.7 0.71428571 0.72857143 0.74285714 0.75714286 0.77142857 0.78571429 0.8 0.81428571 0.82857143 0.84285714 0.85714286 0.87142857 0.88571429 0.9 0.91428571 0.92857143 0.94285714 0.95714286 0.97142857 0.98571429 1 1 1 1 1 1
  arc A45 (-25.601, 14.9902) -> (-26.8439, 16.4344) centre (-45.4614, -0.8441) ccw
  spline S23 degree 5 poles (-26.8439, 16.4344) (-26.8589, 16.4323) (-26.8889, 16.4279) (-26.9339, 16.4213) (-26.9938, 16.4122) (-27.0685, 16.4004) (-27.143, 16.3883) (-27.2173, 16.3758) (-27.2915, 16.3629) (-27.3654, 16.3497) (-27.4392, 16.336) (-27.5127, 16.322) (-27.5861, 16.3076) (-27.6592, 16.2928) (-27.7322, 16.2776) (-27.8049, 16.262) (-27.8774, 16.2461) (-27.9497, 16.2297) (-28.0218, 16.213) (-28.0937, 16.1958) (-28.1653, 16.1783) (-28.2368, 16.1603) (-28.308, 16.142) (-28.3789, 16.1233) (-28.4496, 16.1041) (-28.5201, 16.0846) (-28.5903, 16.0646) (-28.6603, 16.0443) (-28.7301, 16.0235) (-28.7996, 16.0024) (-28.8688, 15.9808) (-28.9377, 15.9588) (-29.0064, 15.9364) (-29.0748, 15.9135) (-29.143, 15.8903) (-29.2108, 15.8666) (-29.2784, 15.8425) (-29.3456, 15.818) (-29.4126, 15.793) (-29.4793, 15.7676) (-29.5457, 15.7418) (-29.6117, 15.7155) (-29.6774, 15.6888) (-29.7428, 15.6616) (-29.8079, 15.634) (-29.8726, 15.6059) (-29.937, 15.5773) (-30.001, 15.5483) (-30.0647, 15.5188) (-30.128, 15.4889) (-30.1909, 15.4584) (-30.2535, 15.4275) (-30.3155, 15.396) (-30.3772, 15.3639) (-30.4384, 15.3314) (-30.4992, 15.2983) (-30.5596, 15.2648) (-30.6196, 15.2307) (-30.6792, 15.1962) (-30.7383, 15.1612) (-30.7968, 15.1255) (-30.8547, 15.089) (-30.9118, 15.0517) (-30.9682, 15.0136) (-31.0239, 14.9747) (-31.0791, 14.9354) (-31.1339, 14.8956) (-31.1884, 14.8555) (-31.2423, 14.8148) (-31.2953, 14.7732) (-31.3467, 14.7299) (-31.386, 14.6935) (-31.4143, 14.665) (-31.4326, 14.6454) (-31.4417, 14.6354) knots -1 -1 -1 -1 -1 -1 -0.98571429 -0.97142857 -0.95714286 -0.94285714 -0.92857143 -0.91428571 -0.9 -0.88571429 -0.87142857 -0.85714286 -0.84285714 -0.82857143 -0.81428571 -0.8 -0.78571429 -0.77142857 -0.75714286 -0.74285714 -0.72857143 -0.71428571 -0.7 -0.68571429 -0.67142857 -0.65714286 -0.64285714 -0.62857143 -0.61428571 -0.6 -0.58571429 -0.57142857 -0.55714286 -0.54285714 -0.52857143 -0.51428571 -0.5 -0.48571429 -0.47142857 -0.45714286 -0.44285714 -0.42857143 -0.41428571 -0.4 -0.38571429 -0.37142857 -0.35714286 -0.34285714 -0.32857143 -0.31428571 -0.3 -0.28571429 -0.27142857 -0.25714286 -0.24285714 -0.22857143 -0.21428571 -0.2 -0.18571429 -0.17142857 -0.15714286 -0.14285714 -0.12857143 -0.11428571 -0.1 -0.08571429 -0.07142857 -0.05714286 -0.04285714 -0.02857143 -0.01428571 0 0 0 0 0 0
  line L25 (-31.4417, 14.6354) -> (-32.1113, 13.8967)
  arc A46 (-34.2561, 13.7053) -> (-32.1113, 13.8967) centre (-33.2874, 14.963) ccw
  arc A47 (-34.2561, 13.7053) -> (-34.8612, 14.1518) centre (-45.4614, -0.8441) ccw
  arc A48 (-35.3981, 14.8093) -> (-34.8612, 14.1518) centre (-33.9448, 15.4482) ccw
  line L26 (-35.3981, 14.8093) -> (-33.2667, 19.4605)
  line L27 (-33.2667, 19.4605) -> (-34.2844, 20.5142)
  spline S24 degree 5 poles (-34.2844, 20.5142) (-34.2847, 20.5222) (-34.2856, 20.5448) (-34.2873, 20.5821) (-34.2898, 20.6341) (-34.2933, 20.7009) (-34.2977, 20.7746) (-34.3025, 20.8483) (-34.3077, 20.9221) (-34.3134, 20.996) (-34.3195, 21.0701) (-34.3261, 21.1441) (-34.3331, 21.2183) (-34.3405, 21.2926) (-34.3483, 21.3669) (-34.3566, 21.4413) (-34.3653, 21.5158) (-34.3744, 21.5904) (-34.384, 21.665) (-34.3939, 21.7397) (-34.4043, 21.8145) (-34.4151, 21.8893) (-34.4241, 21.9492) (-34.431, 21.9942) (-34.4357, 22.0242) (-34.4381, 22.0392) knots 0.70654 0.70654 0.70654 0.70654 0.70654 0.70654 0.714286 0.728571 0.742857 0.757143 0.771429 0.785714 0.8 0.814286 0.828571 0.842857 0.857143 0.871429 0.885714 0.9 0.914286 0.928571 0.942857 0.957143 0.971429 0.985714 1 1 1 1 1 1
  arc A49 (-34.4381, 22.0392) -> (-36.1845, 22.8011) centre (-45.4614, -0.8441) ccw
  spline S25 degree 5 poles (-36.1845, 22.8011) (-36.1971, 22.7927) (-36.2223, 22.7757) (-36.2596, 22.7504) (-36.2968, 22.725) (-36.3338, 22.6995) (-36.3583, 22.6825) (-36.3704, 22.6741) knots -1 -1 -1 -1 -1 -1 -0.985714 -0.971429 -0.957523 -0.957523 -0.957523 -0.957523 -0.957523 -0.957523
  line L28 (-36.3704, 22.6741) -> (-49.1726, 35.9298)
  line L29 (-49.1726, 35.9298) -> (-55.9036, 35.9298)
  line L30 (-49.1726, 17.3449) -> (-49.1726, 18.5703)
  line L31 (-49.1726, 18.5703) -> (-48.6457, 18.4228)
  arc A50 (-49.1726, 17.3449) -> (-48.6457, 18.4228) centre (-50.2296, 18.5294) ccw
  circle A51 centre (-48.6457, 18.4228) radius 2.3821
  constraint coincident L31.end A50.end
extrude "Extrude7" add sketch "Sketch16" against normal blind 12.7 separate body contours A51 sketch seen with x (0.965926, -0.258819, 0) y (0.258819, 0.965926, 0) z (0, 0, 1) at (44.1308, -10.9509, 0) makes body 4 in component "Spur Gear (14 teeth) (1)"
component "Spur Gear (14 teeth)" placed x (1, 0, 0) y (0, 1, 0) z (0, 0, 1) at (0, 0, 0)
component "Spur Gear (14 teeth) (1)" placed x (0.965926, 0.258819, 0) y (-0.258819, 0.965926, 0) z (0, 0, 1) at (-45.4614, -0.8441, 0)
equation "d31 = ( 3 / 4 ) * 1 in"
equation "d32 = ( 3 / 4 ) * 1 in"
equation "d37 = ( 3 / 4 ) * 1 in"
equation "d38 = ( 3 / 4 ) * 1 in"
